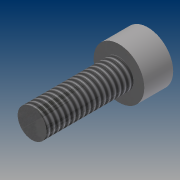
# Autodesk Inventor part: M4_12mm
Saved by Autodesk Inventor 2015 SP1 (Build 190203100, 203)
## iProperties
Created: 2015-03-31
Part Number: M4_12mm
Material: Steel, Alloy
Document SubType Name: Modeling
Designer: nfitch
Mass: 1.96705 g
Surface Area: 2.65465 cm^2
Volume: 0.254469 cm^3
Density: 7.73 g/cm^3
Appearance: Semi-Polished
Author: nfitch
Autodesk Inventor part; units mm, degrees
ref_plane "YZ Plane" through (0, 0, 0) normal (1, 0, 0) x (0, 1, 0)
ref_plane "XZ Plane" through (0, 0, 0) normal (0, 1, 0) x (-1, 0, 0)
ref_plane "XY Plane" through (0, 0, 0) normal (0, 0, 1) x (1, 0, 0)
sketch "Sketch1" plane through (0, 0, 0) normal (0, 1, 0) x (-1, 0, 0)
  circle A0 centre (0, 0) radius 2
  dimension "d0" = 4
  constraints: 1 centre point, 1 coincident
  measures "d0" diameter of A0
extrude "Extrusion1" add sketch "Sketch1" along normal blind 12
sketch "Sketch2" plane through (0, 12, 0) normal (0, 1, 0) x (1, 0, 0)
  circle A0 centre (0, 0) radius 3.5
  dimension "d5" = 7
  constraints: 1 centre point, 1 coincident
  measures "d5" diameter of A0
thread "Thread1" size "M4x0.7" class "6g" standard "ANSI Metric M Profile" full length
extrude "Extrusion2" add sketch "Sketch2" along normal blind 4
sketch "Sketch3" plane through (0, 16, 0) normal (0, 1, 0) x (1, 0, 0)
  circle A0 centre (0, 0) radius 3.5 projected
  circle A1 centre (0, 0) radius 2 projected
  line L0 (-1.7603, 0.9494) -> (-0.058, 1.9992)
  line L1 (-0.058, 1.9992) -> (1.7023, 1.0498)
  line L2 (1.7023, 1.0498) -> (1.7603, -0.9494)
  line L3 (1.7603, -0.9494) -> (0.058, -1.9992)
  line L4 (0.058, -1.9992) -> (-1.7023, -1.0498)
  line L5 (-1.7023, -1.0498) -> (-1.7603, 0.9494)
  constraints: 12 end point, 1 coincident, 15 other
extrude "Extrusion3" cut sketch "Sketch3" against normal blind 3 contours L2 L3 L4 L5 L0 L1
body "Solid1"
